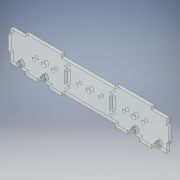
# Autodesk Inventor part: Soporte_Opuesto
Saved by Autodesk Inventor 2019 (Build 230136000, 136)
## iProperties
Created: 2020-04-02
Part Number: Soporte_Opuesto
Material: Generic
Document SubType Name: Modeling
Designer: Jurgen
Density: 1 g/cm^3
Appearance: Clear
Author: Jurgen
Autodesk Inventor part; units mm, degrees
ref_plane "YZ Plane" through (0, 0, 0) normal (1, 0, 0) x (0, 1, 0)
ref_plane "XZ Plane" through (0, 0, 0) normal (0, 1, 0) x (-1, 0, 0)
ref_plane "XY Plane" through (0, 0, 0) normal (0, 0, 1) x (1, 0, 0)
sketch "Sketch1" plane through (0, 0, 0) normal (0, 0, 1) x (1, 0, 0)
  arc A0 (19, -20) -> (20, -19) centre (19, -19) ccw construction
  line L0 (20, -19) -> (20, 19) construction
  arc A1 (20, 19) -> (19, 20) centre (19, 19) ccw construction
  line L1 (19, 20) -> (-19, 20) construction
  arc A2 (-19, 20) -> (-20, 19) centre (-19, 19) ccw construction
  line L2 (-20, 19) -> (-20, -19) construction
  arc A3 (-20, -19) -> (-19, -20) centre (-19, -19) ccw construction
  line L3 (-19, -20) -> (19, -20) construction
  circle A4 centre (-15.5, -15.5) radius 2 construction
  circle A5 centre (15.5, -15.5) radius 2.2846 construction
  circle A6 centre (15.5, 15.5) radius 2 construction
  circle A7 centre (-15.5, 15.5) radius 2 construction
  circle A8 centre (0, 0) radius 11 construction
  line L4 (150, -20) -> (150, 20)
  line L5 (150, 20) -> (-150, 20)
  line L6 (-150, 20) -> (-150, -20)
  line L7 (-150, -20) -> (150, 20) construction
  line L8 (150, -20) -> (-150, 20) construction
  line L9 (50, -20) -> (100, -20) construction
  line L10 (100, -20) -> (100, -25)
  line L11 (100, -25) -> (50, -25)
  line L12 (50, -25) -> (50, -20)
  line L13 (100, -20) -> (150, -20)
  line L14 (-150, -20) -> (50, -20) construction
  line L15 (-150, -20) -> (-100, -20)
  line L16 (-100, -20) -> (-100, -25)
  line L17 (-100, -25) -> (-50, -25)
  line L18 (-50, -25) -> (-50, -20)
  line L19 (-50, -20) -> (50, -20)
  circle A9 centre (-91, 0) radius 3
  circle A10 centre (-59, 0) radius 3
  circle A11 centre (59, 0) radius 3
  circle A12 centre (91, 0) radius 3
  arc A13 (20.5788, -4.4246) -> (20.5788, 4.4246) centre (18.25, 0) ccw construction
  line L20 (6.2877, 11.9463) -> (20.5788, 4.4246) construction
  arc A14 (6.2877, 11.9463) -> (-6.2877, 11.9463) centre (0, 0) ccw construction
  line L21 (-20.5788, 4.4246) -> (-6.2877, 11.9463) construction
  arc A15 (-20.5788, 4.4246) -> (-20.5788, -4.4246) centre (-18.25, 0) ccw construction
  line L22 (-6.2877, -11.9463) -> (-20.5788, -4.4246) construction
  arc A16 (-6.2877, -11.9463) -> (6.2877, -11.9463) centre (0, 0) ccw construction
  line L23 (20.5788, -4.4246) -> (6.2877, -11.9463) construction
  circle A17 centre (18.25, 0) radius 2.5
  circle A18 centre (-18.25, 0) radius 2.5
  line L24 (-5.4726, 10.3977) -> (-17.0094, 4.3256) construction
  arc A19 (5.4726, 10.3977) -> (-5.4726, 10.3977) centre (0, 0) ccw construction
  line L25 (17.0094, 4.3256) -> (5.4726, 10.3977) construction
  arc A20 (17.0094, 4.3256) -> (17.0094, -4.3256) centre (18.25, 0) ccw construction
  line L26 (5.4726, -10.3977) -> (17.0094, -4.3256) construction
  arc A21 (-5.4726, -10.3977) -> (5.4726, -10.3977) centre (0, 0) ccw construction
  line L27 (-17.0094, -4.3256) -> (-5.4726, -10.3977) construction
  arc A22 (-17.0094, -4.3256) -> (-17.0094, 4.3256) centre (-18.25, 0) ccw construction
  circle A23 centre (-75, 0) radius 4
  circle A24 centre (75, 0) radius 4
  dimension "d1" = 50
  dimension "d2" = 5
  dimension "d3" = 50
  dimension "d4" = 50
  dimension "d5" = 50
  dimension "d6" = 6
  dimension "d7" = 6
  dimension "d8" = 32
  dimension "d9" = 6
  dimension "d10" = 6
  dimension "d11" = 32
  dimension "d12" = 59
  dimension "d13" = 59
  dimension "d16" = 8
  dimension "d17" = 16
  dimension "d18" = 8
  dimension "d19" = 16
  dimension "d29" = 100
  dimension "d30" = 40
  dimension "d31" = 40
  constraints: 56 end point, 25 centre point, 24 point on circle, 5 perpendicular, 3 midpoint, 3 parallel, 2 horizontal, 2 point on line, 1 collinear, 1 vertical, 1 other
  measures "d1" distance of L10.end L11.end
  measures "d2" distance of L9.end L10.end
  measures "d3" distance between parallel lines of L4 L10
  measures "d4" distance of L6.end L15.end
  measures "d5" distance of L16.end L17.end
  measures "d6" diameter of A9
  measures "d7" diameter of A10
  measures "d8" distance of A10.centre A9.centre
  measures "d9" diameter of A11
  measures "d10" diameter of A12
  measures "d11" distance of A12.centre A11.centre
  measures "d12" distance of point (0, 0) A10.centre
  measures "d13" distance of point (0, 0) A11.centre
  measures "d16" diameter of A23
  measures "d17" distance of A10.centre A23.centre
  measures "d18" diameter of A24
  measures "d19" distance of A12.centre A24.centre
  measures "d29" distance between parallel lines of L12 L18
  measures "d30" distance of L4.start L4.end
  measures "d31" distance of L5.end L6.end
extrude "Extrusion2" add sketch "Sketch1" along normal blind 5
sketch "Sketch2" plane through (0, 0, 0) normal (0, 0, -1) x (-1, 0, 0)
  circle A0 centre (0, 0) radius 4
  dimension "d22" = 8
  constraints: 1 centre point, 1 coincident
  measures "d22" diameter of A0
extrude "Extrusion3" cut sketch "Sketch2" against normal blind 5
sketch "Sketch3" plane through (-100, -25, 0) normal (0, -1, 0) x (1, 0, 0)
  line L0 (50, 0) -> (0, 0) projected
  line L1 (50, 0) -> (50, 5) projected
  line L2 (0, 5) -> (50, 5) projected
  line L3 (0, 0) -> (0, 5) projected
  line L4 (200, 0) -> (150, 0) projected
  line L5 (200, 0) -> (200, 5) projected
  line L6 (150, 5) -> (200, 5) projected
  line L7 (150, 0) -> (150, 5) projected
  point P0 (100, 0)
extrude "Extrusion4" add sketch "Sketch3" along normal blind 5
sketch "Sketch4" plane through (-50, -20, 0) normal (0, -1, 0) x (1, 0, 0)
  line L0 (-50, 0) -> (-100, 0) projected
  line L1 (-50, 0) -> (-50, 5) projected
  line L2 (-100, 5) -> (-50, 5) projected
  line L3 (-100, 0) -> (-100, 5) projected
  line L4 (100, 0) -> (0, 0) projected
  line L5 (100, 0) -> (100, 5) projected
  line L6 (0, 5) -> (100, 5) projected
  line L7 (0, 0) -> (0, 5) projected
  line L8 (200, 0) -> (150, 0) projected
  line L9 (200, 0) -> (200, 5) projected
  line L10 (150, 5) -> (200, 5) projected
  line L11 (150, 0) -> (150, 5) projected
  point P0 (50, 0)
extrude "Extrusion5" add sketch "Sketch4" along normal blind 5
sketch "Sketch5" plane through (0, 0, 5) normal (0, 0, 1) x (1, 0, 0)
  circle A0 centre (0, 0) radius 4 construction
  circle A1 centre (75, 0) radius 4 construction
  circle A2 centre (-75, 0) radius 4 construction
  circle A3 centre (91, 0) radius 3 construction
  circle A4 centre (59, 0) radius 3 construction
  circle A5 centre (-59, 0) radius 3 construction
  circle A6 centre (-91, 0) radius 3 construction
  circle A7 centre (-18.25, 0) radius 2.5 construction
  circle A8 centre (18.25, 0) radius 2.5 construction
  line L0 (150, 20) -> (150, -25) construction
  line L1 (150, 20) -> (-150, 20) construction
  line L2 (-150, 20) -> (-150, -25) construction
  line L3 (-100, -25) -> (-150, -25) construction
  line L4 (-100, -25) -> (-100, -30) construction
  line L5 (-50, -30) -> (-100, -30) construction
  line L6 (-50, -25) -> (-50, -30) construction
  line L7 (50, -25) -> (-50, -25) construction
  line L8 (50, -25) -> (50, -30) construction
  line L9 (100, -30) -> (50, -30) construction
  line L10 (100, -25) -> (100, -30) construction
  line L11 (150, -25) -> (100, -25) construction
  line L12 (150, 20) -> (-150, 20) projected
  line L13 (-150, 20) -> (-130, 20)
  line L14 (-130, 20) -> (-130, -25)
  line L15 (-130, -25) -> (-150, -25)
  line L16 (-150, -25) -> (-150, 20)
  line L17 (100, -25) -> (150, -25) projected
  line L18 (150, 20) -> (130, 20)
  line L19 (130, 20) -> (130, -25)
  line L20 (130, -25) -> (150, -25)
  line L21 (150, -25) -> (150, 20)
  dimension "d32" = 20
  dimension "d33" = 20
  constraints: 16 end point, 4 parallel, 2 horizontal, 2 perpendicular, 2 point on line
  measures "d32" distance of L14.end L15.end
  measures "d33" distance of L20.end L19.end
extrude "Extrusion6" cut sketch "Sketch5" against normal blind 5
sketch "Sketch6" plane through (0, 0, 5) normal (0, 0, 1) x (1, 0, 0)
  line L0 (-130, 20) -> (-130, -25) construction
  line L1 (-100, -25) -> (-130, -25) construction
  line L2 (-100, -25) -> (-100, -30) construction
  line L3 (-50, -30) -> (-100, -30) construction
  line L4 (-50, -25) -> (-50, -30) construction
  line L5 (50, -25) -> (-50, -25) construction
  line L6 (50, -25) -> (50, -30) construction
  line L7 (100, -30) -> (50, -30) construction
  line L8 (100, -25) -> (100, -30) construction
  line L9 (130, -25) -> (100, -25) construction
  line L10 (130, -25) -> (130, 20) construction
  line L11 (130, 20) -> (-130, 20) construction
  circle A0 centre (0, 0) radius 4 construction
  circle A1 centre (75, 0) radius 4 construction
  circle A2 centre (-75, 0) radius 4 construction
  circle A3 centre (91, 0) radius 3 construction
  circle A4 centre (59, 0) radius 3 construction
  circle A5 centre (-59, 0) radius 3 construction
  circle A6 centre (-91, 0) radius 3 construction
  circle A7 centre (-18.25, 0) radius 2.5 construction
  circle A8 centre (18.25, 0) radius 2.5 construction
  line L12 (-130, 20) -> (130, 20) construction
  line L13 (130, 20) -> (130, 25) construction
  line L14 (130, 25) -> (-130, 25) construction
  line L15 (-130, 25) -> (-130, 20) construction
  line L16 (-100, 25) -> (-50, 25) construction
  line L17 (-50, 25) -> (-50, 30) construction
  line L18 (-50, 30) -> (-100, 30) construction
  line L19 (-100, 30) -> (-100, 25) construction
  line L20 (50, 25) -> (100, 25) construction
  line L21 (100, 25) -> (100, 30) construction
  line L22 (100, 30) -> (50, 30) construction
  line L23 (50, 30) -> (50, 25) construction
  line L24 (130, 20) -> (-130, 20) projected
  line L25 (-130, 20) -> (130, 20)
  line L26 (130, 20) -> (130, 25)
  line L27 (130, 25) -> (100, 25)
  line L28 (100, 25) -> (100, 30)
  line L29 (100, 30) -> (50, 30)
  line L30 (50, 30) -> (50, 25)
  line L31 (50, 25) -> (-50, 25)
  line L32 (-50, 25) -> (-50, 30)
  line L33 (-50, 30) -> (-100, 30)
  line L34 (-100, 30) -> (-100, 25)
  line L35 (-100, 25) -> (-130, 25)
  line L36 (-130, 20) -> (-130, 25)
  dimension "d36" = 5
  dimension "d37" = 5
  dimension "d38" = 5
  constraints: 48 end point, 12 perpendicular, 6 parallel, 4 horizontal, 2 collinear, 2 point on line
  measures "d36" distance of L13.end L12.end
  measures "d37" distance of L17.end L16.end
  measures "d38" distance of L21.end L20.end
extrude "Extrusion7" add sketch "Sketch6" against normal blind 5
sketch "Sketch8" plane through (0, 0, 5) normal (0, 0, 1) x (1, 0, 0)
  line L0 (-130, 25) -> (-130, -25) construction
  line L1 (-100, -25) -> (-130, -25) construction
  line L2 (-100, -25) -> (-100, -30) construction
  line L3 (-50, -30) -> (-100, -30) construction
  line L4 (-50, -25) -> (-50, -30) construction
  line L5 (50, -25) -> (-50, -25) construction
  line L6 (50, -25) -> (50, -30) construction
  line L7 (100, -30) -> (50, -30) construction
  line L8 (100, -25) -> (100, -30) construction
  line L9 (130, -25) -> (100, -25) construction
  line L10 (130, -25) -> (130, 25) construction
  line L11 (130, 25) -> (100, 25) construction
  line L12 (100, 25) -> (100, 30) construction
  line L13 (100, 30) -> (50, 30) construction
  line L14 (50, 30) -> (50, 25) construction
  line L15 (50, 25) -> (-50, 25) construction
  line L16 (-50, 25) -> (-50, 30) construction
  line L17 (-50, 30) -> (-100, 30) construction
  line L18 (-100, 30) -> (-100, 25) projected
  line L19 (-100, 25) -> (-130, 25) construction
  circle A0 centre (0, 0) radius 4 construction
  circle A1 centre (75, 0) radius 4 construction
  circle A2 centre (-75, 0) radius 4 construction
  circle A3 centre (91, 0) radius 3 construction
  circle A4 centre (59, 0) radius 3 construction
  circle A5 centre (-59, 0) radius 3 construction
  circle A6 centre (-91, 0) radius 3 construction
  circle A7 centre (-18.25, 0) radius 2.5 construction
  circle A8 centre (18.25, 0) radius 2.5 construction
  line L20 (-100, 25) -> (-105, 25)
  line L21 (-105, 25) -> (-105, 30)
  line L22 (-105, 30) -> (-100, 30)
  line L23 (-100, 30) -> (-100, 25)
  line L24 (-50, 25) -> (-45, 25)
  line L25 (-45, 25) -> (-45, 30)
  line L26 (-45, 30) -> (-50, 30)
  line L27 (-50, 30) -> (-50, 25)
  line L28 (-100, -25) -> (-130, -25) construction
  line L29 (-100, -25) -> (-105, -25)
  line L30 (-105, -25) -> (-105, -30)
  line L31 (-105, -30) -> (-100, -30)
  line L32 (-100, -30) -> (-100, -25)
  line L33 (-50, -25) -> (50, -25) construction
  line L34 (-50, -25) -> (-45, -25)
  line L35 (-45, -25) -> (-45, -30)
  line L36 (-45, -30) -> (-50, -30)
  line L37 (-50, -30) -> (-50, -25)
  line L38 (50, -25) -> (45, -25)
  line L39 (45, -25) -> (45, -30)
  line L40 (45, -30) -> (50, -30)
  line L41 (50, -30) -> (50, -25)
  line L42 (50, 25) -> (45, 25)
  line L43 (45, 25) -> (45, 30)
  line L44 (45, 30) -> (50, 30)
  line L45 (50, 30) -> (50, 25)
  line L46 (100, 25) -> (105, 25)
  line L47 (105, 25) -> (105, 30)
  line L48 (105, 30) -> (100, 30)
  line L49 (100, 30) -> (100, 25)
  line L50 (130, -25) -> (100, -25) projected
  line L51 (100, -25) -> (105, -25)
  line L52 (105, -25) -> (105, -30)
  line L53 (105, -30) -> (100, -30)
  line L54 (100, -30) -> (100, -25)
  dimension "d43" = 5
  dimension "d44" = 5
  dimension "d45" = 5
  dimension "d46" = 5
  constraints: 64 end point, 16 parallel, 8 horizontal, 8 perpendicular, 6 point on line
  measures "d43" distance of L21.end L22.end
  measures "d44" distance of L26.end L25.end
  measures "d45" distance of L40.end L39.end
  measures "d46" distance of L48.end L47.end
extrude "Extrusion9" add sketch "Sketch8" against normal blind 5
sketch "Sketch9" plane through (0, 0, 5) normal (0, 0, 1) x (1, 0, 0)
  line L0 (-130, 25) -> (-130, -25) construction
  line L1 (-105, -25) -> (-130, -25) construction
  line L2 (-105, -25) -> (-105, -30) construction
  line L3 (-45, -30) -> (-105, -30) construction
  line L4 (-45, -25) -> (-45, -30) construction
  line L5 (45, -25) -> (-45, -25) construction
  line L6 (45, -25) -> (45, -30) construction
  line L7 (105, -30) -> (45, -30) construction
  line L8 (105, -25) -> (105, -30) construction
  line L9 (130, -25) -> (105, -25) construction
  line L10 (130, -25) -> (130, 25) construction
  line L11 (130, 25) -> (105, 25) construction
  line L12 (105, 25) -> (105, 30) construction
  line L13 (105, 30) -> (45, 30) construction
  line L14 (45, 25) -> (45, 30) construction
  line L15 (45, 25) -> (-45, 25) construction
  line L16 (-45, 25) -> (-45, 30) construction
  line L17 (-45, 30) -> (-105, 30) construction
  line L18 (-105, 25) -> (-105, 30) construction
  line L19 (-105, 25) -> (-130, 25) construction
  circle A0 centre (0, 0) radius 4 construction
  circle A1 centre (75, 0) radius 4 construction
  circle A2 centre (-75, 0) radius 4 construction
  circle A3 centre (91, 0) radius 3 construction
  circle A4 centre (59, 0) radius 3 construction
  circle A5 centre (-59, 0) radius 3 construction
  circle A6 centre (-91, 0) radius 3 construction
  circle A7 centre (-18.25, 0) radius 2.5 construction
  circle A8 centre (18.25, 0) radius 2.5 construction
  line L20 (-105, -30) -> (-85, -30) construction
  line L21 (-45, -30) -> (-105, -30) construction
  line L22 (-85, -30) -> (-65, -30)
  line L23 (-65, -30) -> (-65, -25)
  line L24 (-85, -25) -> (-85, -30)
  line L25 (105, -30) -> (85, -30) construction
  line L26 (105, -30) -> (45, -30) construction
  line L27 (85, -30) -> (65, -30)
  line L28 (65, -30) -> (65, -25)
  line L29 (85, -25) -> (85, -30)
  line L30 (-130, 30) -> (-130, -25) construction
  line L31 (-105, -25) -> (-130, -25) construction
  line L32 (-105, -30) -> (-105, -25) construction
  line L33 (-85, -30) -> (-105, -30) construction
  line L34 (-85, -25) -> (-85, -30) construction
  line L35 (-65, -25) -> (-65, -30) construction
  line L36 (-65, -30) -> (-45, -30) construction
  line L37 (-45, -30) -> (-45, -25) construction
  line L38 (45, -25) -> (-45, -25) construction
  line L39 (45, -30) -> (45, -25) construction
  line L40 (65, -30) -> (45, -30) construction
  line L41 (65, -25) -> (65, -30) construction
  line L42 (85, -25) -> (85, -30) construction
  line L43 (85, -30) -> (105, -30) construction
  line L44 (105, -30) -> (105, -25) construction
  line L45 (130, -25) -> (105, -25) construction
  line L46 (130, -25) -> (130, 30) construction
  line L47 (130, 30) -> (105, 30) construction
  line L48 (105, 30) -> (105, 35) construction
  line L49 (105, 35) -> (45, 35) construction
  line L50 (45, 35) -> (45, 30) construction
  line L51 (45, 30) -> (-45, 30) construction
  line L52 (-45, 30) -> (-45, 35) construction
  line L53 (-45, 35) -> (-105, 35) construction
  line L54 (-105, 35) -> (-105, 30) construction
  line L55 (-105, 30) -> (-130, 30) construction
  line L56 (-45, -10) -> (-45, 15) construction
  line L57 (-45, 15) -> (-40, 15) construction
  line L58 (-40, 15) -> (-40, -10) construction
  line L59 (-40, -10) -> (-45, -10) construction
  line L60 (45, 15) -> (45, -10) construction
  line L61 (45, -10) -> (40, -10) construction
  line L62 (40, -10) -> (40, 15) construction
  line L63 (40, 15) -> (45, 15) construction
  circle A9 centre (0, 0) radius 11 construction
  circle A10 centre (75, 0) radius 4 construction
  circle A11 centre (-75, 0) radius 4 construction
  circle A12 centre (91, 0) radius 3 construction
  circle A13 centre (59, 0) radius 3 construction
  circle A14 centre (-59, 0) radius 3 construction
  circle A15 centre (-91, 0) radius 3 construction
  circle A16 centre (15.5, -15.5) radius 2.2846 construction
  circle A17 centre (-15.5, 15.5) radius 2 construction
  circle A18 centre (15.5, 15.5) radius 2 construction
  circle A19 centre (-15.5, -15.5) radius 2 construction
  line L64 (-85, -25) -> (-77, -25) construction
  line L65 (-77, -25) -> (-73, -25) construction
  line L66 (-73, -25) -> (-73, -15) construction
  line L67 (-73, -15) -> (-77, -15) construction
  line L68 (-77, -15) -> (-77, -25) construction
  line L69 (-75, -15) -> (-75, -25) construction
  line L70 (-71, -22) -> (-79, -22) construction
  line L71 (-79, -22) -> (-79, -18) construction
  line L72 (-79, -18) -> (-71, -18) construction
  line L73 (-71, -18) -> (-71, -22) construction
  line L74 (-71, -22) -> (-79, -18) construction
  line L75 (-79, -22) -> (-71, -18) construction
  line L76 (-77, -25) -> (-77, -22)
  line L77 (-77, -22) -> (-79, -22)
  line L78 (-79, -22) -> (-79, -18)
  line L79 (-79, -18) -> (-77, -18)
  line L80 (-77, -18) -> (-77, -15)
  line L81 (-77, -15) -> (-73, -15)
  line L82 (-73, -15) -> (-73, -18)
  line L83 (-73, -18) -> (-71, -18)
  line L84 (-71, -18) -> (-71, -22)
  line L85 (-71, -22) -> (-73, -22)
  line L86 (-73, -22) -> (-73, -25)
  line L87 (-85, -30) -> (-105, -30) construction
  line L88 (-95, -30) -> (-95, 35) construction
  line L89 (-45, 30) -> (45, 30) construction
  line L90 (0, 30) -> (0, -25) construction
  line L91 (-119, -22) -> (-117, -22)
  line L92 (-113, -22) -> (-111, -22)
  line L93 (-119, -22) -> (-111, -22) construction
  line L94 (-111, -18) -> (-113, -18)
  line L95 (-111, -18) -> (-119, -18) construction
  line L96 (-111, -22) -> (-111, -18) construction
  line L97 (-111, -22) -> (-111, -18)
  line L98 (-111, -22) -> (-119, -18) construction
  line L99 (-119, -22) -> (-111, -18) construction
  line L100 (-117, -25) -> (-117, -15) construction
  line L101 (-113, -15) -> (-113, -25) construction
  line L102 (-115, -15) -> (-115, -25) construction
  line L103 (-117, -18) -> (-119, -18)
  line L104 (-119, -18) -> (-119, -22)
  line L105 (-117, -15) -> (-113, -15) construction
  line L106 (-113, -18) -> (-113, -15)
  line L107 (-117, -15) -> (-117, -18)
  line L108 (-119, -18) -> (-119, -22) construction
  line L109 (-113, -25) -> (-117, -25) construction
  line L110 (-113, -25) -> (-113, -22)
  line L111 (-117, -25) -> (-113, -25)
  line L112 (-117, -22) -> (-117, -25)
  line L113 (-113, -15) -> (-117, -15)
  line L114 (77, -18) -> (77, -15)
  line L115 (77, -15) -> (73, -15)
  line L116 (73, -15) -> (77, -15) construction
  line L117 (73, -15) -> (73, -18)
  line L118 (73, -25) -> (73, -15) construction
  line L119 (75, -15) -> (75, -25) construction
  line L120 (77, -15) -> (77, -25) construction
  line L121 (85, -25) -> (77, -25) construction
  line L122 (113, -25) -> (113, -22)
  line L123 (113, -18) -> (113, -15)
  line L124 (117, -15) -> (117, -18)
  line L125 (117, -15) -> (113, -15) construction
  line L126 (113, -15) -> (117, -15)
  line L127 (111, -18) -> (113, -18)
  line L128 (117, -18) -> (119, -18)
  line L129 (115, -15) -> (115, -25) construction
  line L130 (113, -15) -> (113, -25) construction
  line L131 (117, -25) -> (117, -15) construction
  line L132 (111, -22) -> (111, -18) construction
  line L133 (119, -22) -> (117, -22)
  line L134 (119, -18) -> (119, -22) construction
  line L135 (119, -18) -> (119, -22)
  line L136 (111, -18) -> (119, -18) construction
  line L137 (117, -22) -> (117, -25)
  line L138 (111, -22) -> (119, -18) construction
  line L139 (119, -22) -> (111, -22) construction
  line L140 (119, -22) -> (111, -18) construction
  line L141 (113, -25) -> (117, -25) construction
  line L142 (117, -25) -> (113, -25)
  line L143 (111, -22) -> (111, -18)
  line L144 (113, -22) -> (111, -22)
  line L145 (73, -22) -> (73, -25)
  line L146 (77, -25) -> (77, -22)
  line L147 (77, -22) -> (79, -22)
  line L148 (79, -18) -> (77, -18)
  line L149 (79, -22) -> (79, -18)
  line L150 (79, -22) -> (79, -18) construction
  line L151 (79, -18) -> (71, -18) construction
  line L152 (71, -22) -> (79, -18) construction
  line L153 (71, -22) -> (79, -22) construction
  line L154 (79, -22) -> (71, -18) construction
  line L155 (71, -18) -> (71, -22) construction
  line L156 (73, -18) -> (71, -18)
  line L157 (71, -18) -> (71, -22)
  line L158 (71, -22) -> (73, -22)
  line L159 (-65, -25) -> (-73, -25)
  line L160 (-77, -25) -> (-85, -25)
  line L161 (-65, -25) -> (-73, -25) construction
  line L162 (-75, -25) -> (-85, -25) construction
  line L163 (-65, -25) -> (-73, -25) construction
  line L164 (-75, -25) -> (-85, -25) construction
  line L165 (65, -25) -> (73, -25)
  line L166 (77, -25) -> (85, -25)
  line L167 (85, -25) -> (75, -25) construction
  line L168 (73, -25) -> (65, -25) construction
  point P0 (-75, -20)
  point P1 (-115, -20)
  point P2 (115, -20)
  point P3 (75, -20)
  dimension "d49" = 20
  dimension "d50" = 20
  dimension "d51" = 20
  dimension "d52" = 20
  dimension "d53" = 8
  dimension "d54" = 4
  dimension "d55" = 10
  dimension "d56" = 8
  dimension "d57" = 4
  constraints: 294 end point, 45 symmetric about line, 36 point on line, 14 midpoint, 11 centre point, 10 parallel, 9 perpendicular, 4 horizontal, 3 collinear
  measures "d49" distance of L2.end L20.end
  measures "d50" distance of L24.start L23.end
  measures "d51" distance of L7.start L25.end
  measures "d52" distance of L28.end L29.start
  measures "d53" distance of L34.start L64.end
  measures "d54" distance of L67.end L66.end
  measures "d55" distance of L65.end L66.end
  measures "d56" distance of L71.end L72.end
  measures "d57" distance of L70.end L71.end
extrude "Extrusion10" cut sketch "Sketch9" against normal blind 5
sketch "Sketch10" plane through (0, 0, 5) normal (0, 0, 1) x (1, 0, 0)
  circle A0 centre (18.25, 0) radius 2.5 construction
  circle A1 centre (-18.25, 0) radius 2.5 construction
  circle A2 centre (-91, 0) radius 3 construction
  circle A3 centre (-59, 0) radius 3 construction
  circle A4 centre (59, 0) radius 3 construction
  circle A5 centre (91, 0) radius 3 construction
  circle A6 centre (-75, 0) radius 4 construction
  circle A7 centre (75, 0) radius 4 construction
  circle A8 centre (0, 0) radius 4 construction
  line L0 (-85, -30) -> (-85, -25) construction
  line L1 (-85, -25) -> (-77, -25) construction
  line L2 (-77, -25) -> (-77, -22) construction
  line L3 (-77, -22) -> (-79, -22) construction
  line L4 (-79, -22) -> (-79, -18) construction
  line L5 (-79, -18) -> (-77, -18) construction
  line L6 (-77, -18) -> (-77, -15) construction
  line L7 (-77, -15) -> (-73, -15) construction
  line L8 (-73, -15) -> (-73, -18) construction
  line L9 (-73, -18) -> (-71, -18) construction
  line L10 (-71, -18) -> (-71, -22) construction
  line L11 (-71, -22) -> (-73, -22) construction
  line L12 (-73, -22) -> (-73, -25) construction
  line L13 (-73, -25) -> (-65, -25) construction
  line L14 (-65, -25) -> (-65, -30) construction
  line L15 (-45, -30) -> (-65, -30) construction
  line L16 (-45, -25) -> (-45, -30) construction
  line L17 (45, -25) -> (-45, -25) construction
  line L18 (45, -25) -> (45, -30) construction
  line L19 (65, -30) -> (45, -30) construction
  line L20 (65, -30) -> (65, -25) construction
  line L21 (65, -25) -> (73, -25) construction
  line L22 (73, -25) -> (73, -22) construction
  line L23 (73, -22) -> (71, -22) construction
  line L24 (71, -22) -> (71, -18) construction
  line L25 (71, -18) -> (73, -18) construction
  line L26 (73, -18) -> (73, -15) construction
  line L27 (73, -15) -> (77, -15) construction
  line L28 (77, -15) -> (77, -18) construction
  line L29 (77, -18) -> (79, -18) construction
  line L30 (79, -18) -> (79, -22) construction
  line L31 (79, -22) -> (77, -22) construction
  line L32 (77, -22) -> (77, -25) construction
  line L33 (77, -25) -> (85, -25) construction
  line L34 (85, -25) -> (85, -30) construction
  line L35 (105, -30) -> (85, -30) construction
  line L36 (105, -25) -> (105, -30) construction
  line L37 (113, -25) -> (105, -25) construction
  line L38 (113, -25) -> (113, -22) construction
  line L39 (113, -22) -> (111, -22) construction
  line L40 (111, -22) -> (111, -18) construction
  line L41 (111, -18) -> (113, -18) construction
  line L42 (113, -18) -> (113, -15) construction
  line L43 (113, -15) -> (117, -15) construction
  line L44 (117, -15) -> (117, -18) construction
  line L45 (117, -18) -> (119, -18) construction
  line L46 (119, -18) -> (119, -22) construction
  line L47 (119, -22) -> (117, -22) construction
  line L48 (117, -22) -> (117, -25) construction
  line L49 (130, -25) -> (117, -25) construction
  line L50 (130, -25) -> (130, 25) construction
  line L51 (130, 25) -> (105, 25) construction
  line L52 (105, 25) -> (105, 30) construction
  line L53 (105, 30) -> (45, 30) construction
  line L54 (45, 25) -> (45, 30) construction
  line L55 (45, 25) -> (-45, 25) construction
  line L56 (-45, 25) -> (-45, 30) construction
  line L57 (-45, 30) -> (-105, 30) construction
  line L58 (-105, 25) -> (-105, 30) construction
  line L59 (-105, 25) -> (-130, 25) construction
  line L60 (-130, 25) -> (-130, -25) construction
  line L61 (-117, -25) -> (-130, -25) construction
  line L62 (-117, -25) -> (-117, -22) construction
  line L63 (-117, -22) -> (-119, -22) construction
  line L64 (-119, -22) -> (-119, -18) construction
  line L65 (-119, -18) -> (-117, -18) construction
  line L66 (-117, -18) -> (-117, -15) construction
  line L67 (-117, -15) -> (-113, -15) construction
  line L68 (-113, -15) -> (-113, -18) construction
  line L69 (-113, -18) -> (-111, -18) construction
  line L70 (-111, -18) -> (-111, -22) construction
  line L71 (-111, -22) -> (-113, -22) construction
  line L72 (-113, -22) -> (-113, -25) construction
  line L73 (-105, -25) -> (-113, -25) construction
  line L74 (-105, -25) -> (-105, -30) construction
  line L75 (-85, -30) -> (-105, -30) construction
  line L76 (-130, 0) -> (130, 0) construction
  line L77 (-35, -10) -> (-40, -10)
  line L78 (-40, -10) -> (-40, 10)
  line L79 (-40, 10) -> (-35, 10)
  line L80 (-35, 10) -> (-35, -10)
  line L81 (-35, -10) -> (-40, 10) construction
  line L82 (-40, -10) -> (-35, 10) construction
  line L83 (40, -10) -> (35, -10)
  line L84 (35, -10) -> (35, 10)
  line L85 (35, 10) -> (40, 10)
  line L86 (40, 10) -> (40, -10)
  line L87 (40, -10) -> (35, 10) construction
  line L88 (35, -10) -> (40, 10) construction
  line L89 (0, 25) -> (0, -25) construction
  line L90 (-45, -25) -> (45, -25) construction
  line L91 (-37.5, -25) -> (-37.5, 25) construction
  line L92 (37.5, -25) -> (37.5, 25) construction
  circle A9 centre (-37.5, 16) radius 2
  circle A10 centre (-37.5, -16) radius 2
  circle A11 centre (37.5, 16) radius 2
  circle A12 centre (37.5, -16) radius 2
  point P0 (-37.5, 0)
  point P1 (37.5, 0)
  dimension "d60" = 5
  dimension "d61" = 20
  dimension "d62" = 5
  dimension "d63" = 20
  dimension "d64" = 5
  dimension "d65" = 5
  dimension "d66" = 4
  dimension "d67" = 4
  dimension "d68" = 4
  dimension "d69" = 4
  dimension "d70" = 6
  dimension "d71" = 6
  dimension "d72" = 6
  dimension "d73" = 6
  constraints: 32 end point, 10 point on line, 8 midpoint, 4 centre point, 4 parallel, 4 perpendicular, 2 horizontal
  measures "d60" distance of L78.end L79.end
  measures "d61" distance of L77.end L78.end
  measures "d62" distance of L84.end L85.end
  measures "d63" distance of L83.end L84.end
  measures "d64" distance between parallel lines of L56 L78
  measures "d65" distance between parallel lines of L54 L86
  measures "d66" diameter of A9
  measures "d67" diameter of A10
  measures "d68" diameter of A11
  measures "d69" diameter of A12
  measures "d70" distance from line of L79 A9.centre
  measures "d71" distance from line of A10.centre L77
  measures "d72" distance from line of L85 A11.centre
  measures "d73" distance from line of A12.centre L83
extrude "Extrusion11" cut sketch "Sketch10" against normal blind 10
sketch "Sketch11" plane through (0, 0, 5) normal (0, 0, 1) x (1, 0, 0)
  line L0 (-35, 10) -> (-35, -10) construction
  line L1 (-35, -10) -> (-40, -10) construction
  line L2 (-40, -10) -> (-40, 10) construction
  line L3 (-40, 10) -> (-35, 10) construction
  circle A0 centre (37.5, 16) radius 2 construction
  circle A1 centre (-37.5, 16) radius 2 construction
  circle A2 centre (-37.5, -16) radius 2 construction
  circle A3 centre (37.5, -16) radius 2 construction
  line L4 (40, 10) -> (40, -10) construction
  line L5 (40, -10) -> (35, -10) construction
  line L6 (35, -10) -> (35, 10) construction
  line L7 (35, 10) -> (40, 10) construction
  circle A4 centre (18.25, 0) radius 2.5 construction
  circle A5 centre (-18.25, 0) radius 2.5 construction
  circle A6 centre (-91, 0) radius 3 construction
  circle A7 centre (-59, 0) radius 3 construction
  circle A8 centre (59, 0) radius 3 construction
  circle A9 centre (91, 0) radius 3 construction
  circle A10 centre (-75, 0) radius 4 construction
  circle A11 centre (75, 0) radius 4 construction
  circle A12 centre (0, 0) radius 4 construction
  line L8 (-85, -30) -> (-85, -25) construction
  line L9 (-85, -25) -> (-77, -25) construction
  line L10 (-77, -25) -> (-77, -22) construction
  line L11 (-77, -22) -> (-79, -22) construction
  line L12 (-79, -22) -> (-79, -18) construction
  line L13 (-79, -18) -> (-77, -18) construction
  line L14 (-77, -18) -> (-77, -15) construction
  line L15 (-77, -15) -> (-73, -15) construction
  line L16 (-73, -15) -> (-73, -18) construction
  line L17 (-73, -18) -> (-71, -18) construction
  line L18 (-71, -18) -> (-71, -22) construction
  line L19 (-71, -22) -> (-73, -22) construction
  line L20 (-73, -22) -> (-73, -25) construction
  line L21 (-73, -25) -> (-65, -25) construction
  line L22 (-65, -25) -> (-65, -30) construction
  line L23 (-45, -30) -> (-65, -30) construction
  line L24 (-45, -25) -> (-45, -30) construction
  line L25 (45, -25) -> (-45, -25) construction
  line L26 (45, -25) -> (45, -30) construction
  line L27 (65, -30) -> (45, -30) construction
  line L28 (65, -30) -> (65, -25) construction
  line L29 (65, -25) -> (73, -25) construction
  line L30 (73, -25) -> (73, -22) construction
  line L31 (73, -22) -> (71, -22) construction
  line L32 (71, -22) -> (71, -18) construction
  line L33 (71, -18) -> (73, -18) construction
  line L34 (73, -18) -> (73, -15) construction
  line L35 (73, -15) -> (77, -15) construction
  line L36 (77, -15) -> (77, -18) construction
  line L37 (77, -18) -> (79, -18) construction
  line L38 (79, -18) -> (79, -22) construction
  line L39 (79, -22) -> (77, -22) construction
  line L40 (77, -22) -> (77, -25) construction
  line L41 (77, -25) -> (85, -25) construction
  line L42 (85, -25) -> (85, -30) construction
  line L43 (105, -30) -> (85, -30) construction
  line L44 (105, -25) -> (105, -30) construction
  line L45 (113, -25) -> (105, -25) construction
  line L46 (113, -25) -> (113, -22) construction
  line L47 (113, -22) -> (111, -22) construction
  line L48 (111, -22) -> (111, -18) construction
  line L49 (111, -18) -> (113, -18) construction
  line L50 (113, -18) -> (113, -15) construction
  line L51 (113, -15) -> (117, -15) construction
  line L52 (117, -15) -> (117, -18) construction
  line L53 (117, -18) -> (119, -18) construction
  line L54 (119, -18) -> (119, -22) construction
  line L55 (119, -22) -> (117, -22) construction
  line L56 (117, -22) -> (117, -25) construction
  line L57 (130, -25) -> (117, -25) construction
  line L58 (130, -25) -> (130, 25) construction
  line L59 (130, 25) -> (105, 25) construction
  line L60 (105, 25) -> (105, 30) construction
  line L61 (105, 30) -> (45, 30) construction
  line L62 (45, 25) -> (45, 30) construction
  line L63 (45, 25) -> (-45, 25) construction
  line L64 (-45, 25) -> (-45, 30) construction
  line L65 (-45, 30) -> (-105, 30) construction
  line L66 (-105, 25) -> (-105, 30) construction
  line L67 (-105, 25) -> (-130, 25) construction
  line L68 (-130, 25) -> (-130, -25) construction
  line L69 (-117, -25) -> (-130, -25) construction
  line L70 (-117, -25) -> (-117, -22) construction
  line L71 (-117, -22) -> (-119, -22) construction
  line L72 (-119, -22) -> (-119, -18) construction
  line L73 (-119, -18) -> (-117, -18) construction
  line L74 (-117, -18) -> (-117, -15) construction
  line L75 (-117, -15) -> (-113, -15) construction
  line L76 (-113, -15) -> (-113, -18) construction
  line L77 (-113, -18) -> (-111, -18) construction
  line L78 (-111, -18) -> (-111, -22) construction
  line L79 (-111, -22) -> (-113, -22) construction
  line L80 (-113, -22) -> (-113, -25) construction
  line L81 (-105, -25) -> (-113, -25) construction
  line L82 (-105, -25) -> (-105, -30) construction
  line L83 (-85, -30) -> (-105, -30) construction
  line L84 (-130, 15) -> (-133.5, 15)
  line L85 (-133.5, 15) -> (-133.5, -10)
  line L86 (-133.5, -10) -> (-130, -10)
  line L87 (-130, -10) -> (-130, 15)
  line L88 (45, 25) -> (-45, 25) construction
  line L89 (0, 25) -> (0, -25) construction
  line L90 (45, -25) -> (-45, -25) construction
  line L91 (130, 15) -> (133.5, 15)
  line L92 (133.5, 15) -> (133.5, -10)
  line L93 (133.5, -10) -> (130, -10)
  line L94 (130, -10) -> (130, 15)
  dimension "d76" = 3.5
  dimension "d77" = 25
  dimension "d78" = 10
  constraints: 18 end point, 4 symmetric about line, 2 midpoint, 2 parallel, 1 horizontal, 1 perpendicular, 1 point on line
  measures "d76" distance of L86.end L85.end
  measures "d77" distance of L85.end L84.end
  measures "d78" distance between parallel lines of L67 L84
extrude "Extrusion12" add sketch "Sketch11" against normal blind 5
body "Solid2"
